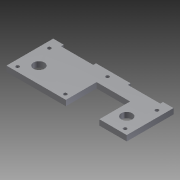
# Autodesk Inventor part: carro x lado polea pieza2
Saved by Autodesk Inventor 2012 (Build 160160000, 160)
## iProperties
Created: 2014-12-16
Part Number: carro x lado polea pieza2
Material: Default
Document SubType Name: Modeling
Designer: PRINCIPAL
Density: 1 g/cm^3
Author: PRINCIPAL
Autodesk Inventor part; units mm, degrees
ref_plane "YZ Plane" through (0, 0, 0) normal (1, 0, 0) x (0, 1, 0)
ref_plane "XZ Plane" through (0, 0, 0) normal (0, 1, 0) x (-1, 0, 0)
ref_plane "XY Plane" through (0, 0, 0) normal (0, 0, 1) x (1, 0, 0)
sketch "Boceto1" plane through (0, 0, 0) normal (0, 0, 1) x (1, 0, 0)
  arc A0 (-116.1173, -7.6512) -> (-117.6673, -9.2012) centre (-116.1173, -9.2012) ccw
  arc A1 (-117.6673, -9.2012) -> (-116.1173, -10.7512) centre (-116.1173, -9.2012) ccw
  arc A2 (-116.1173, -10.7512) -> (-114.5673, -9.2012) centre (-116.1173, -9.2012) ccw
  arc A3 (-114.5673, -9.2012) -> (-116.1173, -7.6512) centre (-116.1173, -9.2012) ccw
  arc A4 (-67.1173, -3.6512) -> (-68.6673, -5.2012) centre (-67.1173, -5.2012) ccw
  arc A5 (-68.6673, -5.2012) -> (-67.1173, -6.7512) centre (-67.1173, -5.2012) ccw
  arc A6 (-67.1173, -6.7512) -> (-65.5673, -5.2012) centre (-67.1173, -5.2012) ccw
  arc A7 (-65.5673, -5.2012) -> (-67.1173, -3.6512) centre (-67.1173, -5.2012) ccw
  arc A8 (-18.1173, -7.6512) -> (-19.6673, -9.2012) centre (-18.1173, -9.2012) ccw
  arc A9 (-19.6673, -9.2012) -> (-18.1173, -10.7512) centre (-18.1173, -9.2012) ccw
  arc A10 (-18.1173, -10.7512) -> (-16.5673, -9.2012) centre (-18.1173, -9.2012) ccw
  arc A11 (-16.5673, -9.2012) -> (-18.1173, -7.6512) centre (-18.1173, -9.2012) ccw
  arc A12 (-72.6173, -36.6512) -> (-74.1673, -38.2012) centre (-72.6173, -38.2012) ccw
  arc A13 (-74.1673, -38.2012) -> (-72.6173, -39.7512) centre (-72.6173, -38.2012) ccw
  arc A14 (-72.6173, -39.7512) -> (-71.0673, -38.2012) centre (-72.6173, -38.2012) ccw
  arc A15 (-71.0673, -38.2012) -> (-72.6173, -36.6512) centre (-72.6173, -38.2012) ccw
  arc A16 (-18.1173, -36.6512) -> (-19.6673, -38.2012) centre (-18.1173, -38.2012) ccw
  arc A17 (-19.6673, -38.2012) -> (-18.1173, -39.7512) centre (-18.1173, -38.2012) ccw
  arc A18 (-18.1173, -39.7512) -> (-16.5673, -38.2012) centre (-18.1173, -38.2012) ccw
  arc A19 (-16.5673, -38.2012) -> (-18.1173, -36.6512) centre (-18.1173, -38.2012) ccw
  arc A20 (-116.1173, -36.6512) -> (-117.6673, -38.2012) centre (-116.1173, -38.2012) ccw
  arc A21 (-117.6673, -38.2012) -> (-116.1173, -39.7512) centre (-116.1173, -38.2012) ccw
  arc A22 (-116.1173, -39.7512) -> (-114.5673, -38.2012) centre (-116.1173, -38.2012) ccw
  arc A23 (-114.5673, -38.2012) -> (-116.1173, -36.6512) centre (-116.1173, -38.2012) ccw
  arc A24 (-107.1173, -22.7512) -> (-112.0673, -27.7012) centre (-107.1173, -27.7012) ccw
  arc A25 (-112.0673, -27.7012) -> (-107.1173, -32.6512) centre (-107.1173, -27.7012) ccw
  arc A26 (-107.1173, -32.6512) -> (-102.1673, -27.7012) centre (-107.1173, -27.7012) ccw
  arc A27 (-102.1673, -27.7012) -> (-107.1173, -22.7512) centre (-107.1173, -27.7012) ccw
  arc A28 (-27.1173, -22.7512) -> (-32.0673, -27.7012) centre (-27.1173, -27.7012) ccw
  arc A29 (-32.0673, -27.7012) -> (-27.1173, -32.6512) centre (-27.1173, -27.7012) ccw
  arc A30 (-27.1173, -32.6512) -> (-22.1673, -27.7012) centre (-27.1173, -27.7012) ccw
  arc A31 (-22.1673, -27.7012) -> (-27.1173, -22.7512) centre (-27.1173, -27.7012) ccw
  line L0 (-67.8173, -14.5012) -> (-37.3173, -14.5012)
  line L1 (-37.3173, -14.5012) -> (-37.3173, -42.5012)
  line L2 (-37.3173, -42.5012) -> (-12.3173, -42.5012)
  line L3 (-12.3173, -42.5012) -> (-12.3173, 0.0988)
  line L4 (-12.3173, 0.0988) -> (-21.9173, 0.0988)
  line L5 (-21.9173, 0.0988) -> (-21.9173, -2.4012)
  line L6 (-21.9173, -2.4012) -> (-51.3173, -2.4012)
  line L7 (-51.3173, -2.4012) -> (-51.3173, 0.0988)
  line L8 (-51.3173, 0.0988) -> (-82.9173, 0.0988)
  line L9 (-82.9173, 0.0988) -> (-82.9173, -2.4012)
  line L10 (-82.9173, -2.4012) -> (-112.3173, -2.4012)
  line L11 (-112.3173, -2.4012) -> (-112.3173, 0.0988)
  line L12 (-112.3173, 0.0988) -> (-121.9173, 0.0988)
  line L13 (-121.9173, 0.0988) -> (-121.9173, -42.5012)
  line L14 (-121.9173, -42.5012) -> (-67.8173, -42.5012)
  line L15 (-67.8173, -42.5012) -> (-67.8173, -14.5012)
  point P0 (0, 0)
  constraints: 64 point on circle, 32 centre point, 32 end point
extrude "Extrusión1" add sketch "Boceto1" along normal blind 5
